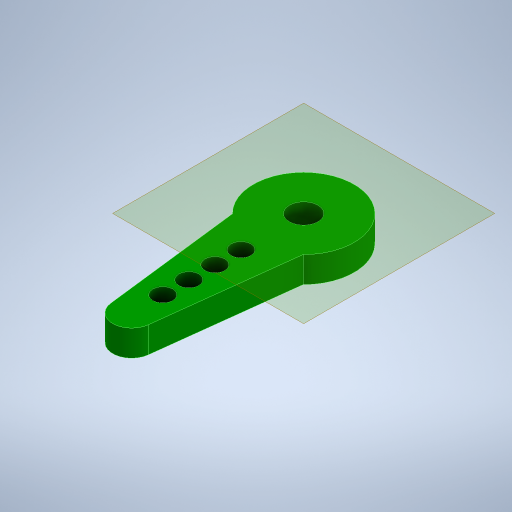
# Autodesk Inventor part: X4_leg_Servo_horn
Saved by Autodesk Inventor 2023.1 (Build 271208000, 208)
## iProperties
Created: 2022-08-18
Part Number: X4_leg_Servo_horn
Material: Default New Material
Document SubType Name: Modeling
Designer: Windows10
Density: 1 g/cm^3
Appearance: Generic
Author: Windows10
Autodesk Inventor part; units mm, degrees
ref_plane "YZ Plane" through (0, 0, 0) normal (1, 0, 0) x (0, 1, 0)
ref_plane "XZ Plane" through (0, 0, 0) normal (0, 1, 0) x (-1, 0, 0)
ref_plane "XY Plane" through (0, 0, 0) normal (0, 0, 1) x (1, 0, 0)
ref_plane "Work Plane12" through (10, 45.7, 9.8) normal (0, -1, 0) x (1, 0, 0)
sketch "Sketch20" plane through (10, 45.7, 9.8) normal (0, -1, 0) x (1, 0, 0)
  circle A0 centre (0, 10.22) radius 1.15 projected
  circle A1 centre (0, 13.22) radius 1.15 projected
  circle A2 centre (0, 7.22) radius 1.15 projected
  circle A3 centre (0, 16.22) radius 1.15 projected
  arc A4 (2.55, 20.12) -> (-2.55, 20.12) centre (0, 19.8141) ccw projected
  line L0 (-2.55, 20.12) -> (-4.4453, 4.3219) projected
  arc A5 (-4.4453, 4.3219) -> (4.4453, 4.3219) centre (0, 0) ccw projected
  line L1 (4.4453, 4.3219) -> (2.55, 20.12) projected
  circle A6 centre (0, 0) radius 1.65 projected
  arc A7 (2.1528, 20.0724) -> (-2.1528, 20.0724) centre (0, 19.8141) ccw
  line L2 (-2.1528, 20.0724) -> (-4.0646, 4.1375)
  arc A8 (-4.0646, 4.1375) -> (4.0646, 4.1375) centre (0, 0) ccw
  line L3 (4.0646, 4.1375) -> (2.1528, 20.0724)
  point P0 (-10, -9.8)
  dimension "d95" = 0.4
  constraints: 4 end point, 4 point on circle, 2 centre point, 3 other
  measures "d95" distance between parallel lines of L1 L3
extrude "Extrusion21" add sketch "Sketch20" along normal blind 3 contours L3 A8 L2 A7
body "Solid11"
